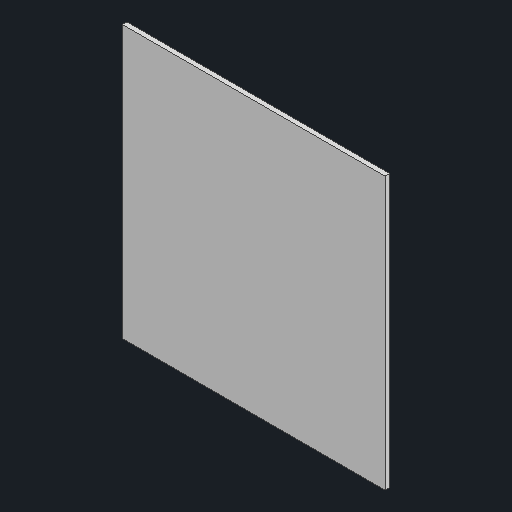
# Autodesk Inventor part: ФАЛЬШБОРТА 2
Saved by Autodesk Inventor 2025 (Build 290162000, 162)
## iProperties
Created: 2025-01-26
Part Number: ФАЛЬШБОРТА 2
Material: Типовые
Document SubType Name: Modeling
Designer: GameHD
Density: 1 g/cm^3
Appearance: По умолчанию
Author: GameHD
Autodesk Inventor part; units mm, degrees
ref_plane "YZ Plane" through (0, 0, 0) normal (1, 0, 0) x (0, 1, 0)
ref_plane "XZ Plane" through (0, 0, 0) normal (0, 1, 0) x (-1, 0, 0)
ref_plane "XY Plane" through (0, 0, 0) normal (0, 0, 1) x (1, 0, 0)
sketch "Эскиз1" plane through (0, 0, 0) normal (0, 0, 1) x (1, 0, 0)
  line L0 (0, 0) -> (230, 0)
  line L1 (230, 0) -> (230, 238)
  line L2 (230, 238) -> (0, 238)
  line L3 (0, 238) -> (0, 0)
  dimension "d0" = 230
  dimension "d1" = 238
  constraints: 8 end point, 2 parallel, 1 horizontal, 1 perpendicular
  measures "d0" distance of L2.end L1.end
  measures "d1" distance of L1.end L0.end
extrude "Выдавливание1" add sketch "Эскиз1" along normal blind 4
